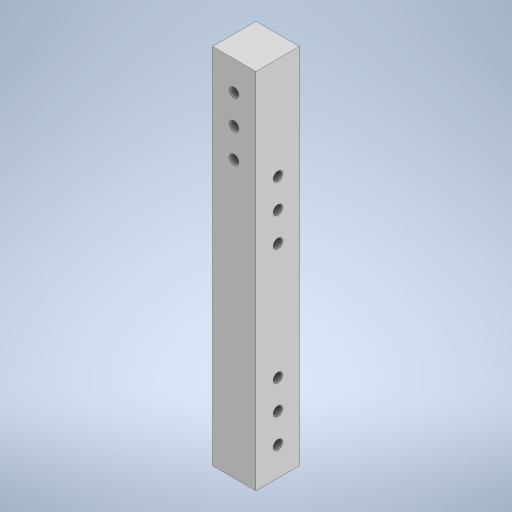
# Autodesk Inventor part: 射出_角柱11
Saved by Autodesk Inventor 2023 (Build 270158000, 158)
## iProperties
Created: 2022-04-20
Part Number: 射出_角柱11
Material: 一般
Document SubType Name: Modeling
Designer: yuta
Density: 1 g/cm^3
Appearance: 既定
Author: yuta
Autodesk Inventor part; units mm, degrees
ref_plane "YZ Plane" through (0, 0, 0) normal (1, 0, 0) x (0, 1, 0)
ref_plane "XZ Plane" through (0, 0, 0) normal (0, 1, 0) x (-1, 0, 0)
ref_plane "XY Plane" through (0, 0, 0) normal (0, 0, 1) x (1, 0, 0)
sketch "スケッチ1" plane through (0, 0, 0) normal (0, 1, 0) x (-1, 0, 0)
  line L0 (0, 0) -> (15, 0)
  line L1 (15, 0) -> (15, -15)
  line L2 (15, -15) -> (0, -15)
  line L3 (0, -15) -> (0, 0)
  dimension "d0" = 15
  dimension "d1" = 15
  constraints: 8 end point, 2 parallel, 1 horizontal, 1 perpendicular
  measures "d0" distance of L1.end L2.end
  measures "d1" distance of L0.end L1.end
extrude "押し出し1" add sketch "スケッチ1" along normal blind 125
sketch "スケッチ2" plane through (-15, 0, 0) normal (0, 0, 1) x (1, 0, 0)
  line L0 (0, 125) -> (15, 125) projected
  line L1 (0, 0) -> (0, 125) projected
  point P0 (15, 0)
  point P1 (7.5, 115)
  point P2 (7.5, 105)
  point P3 (7.5, 95)
  dimension "d4" = 10
  dimension "d5" = 7.5
  dimension "d6" = 7.5
  dimension "d7" = 7.5
  dimension "d8" = 10
  dimension "d9" = 10
  measures "d4" distance from line of L0 point (7.5, 115)
  measures "d5" distance from line of L1 point (7.5, 115)
  measures "d6" distance from line of L1 point (7.5, 105)
  measures "d7" distance from line of L1 point (7.5, 95)
  measures "d8" distance of point (7.5, 105) point (7.5, 115)
  measures "d9" distance of point (7.5, 95) point (7.5, 105)
hole "穴1" at (-7.5, 115, 0) at (-7.5, 105, 0) at (-7.5, 95, 0) direction (0, 0, -1) diameter 3.2 end through all
sketch "スケッチ3" plane through (0, 0, 0) normal (1, 0, 0) x (0, 0, -1)
  line L0 (0, 125) -> (15, 125) projected
  line L1 (15, 0) -> (15, 125) projected
  line L2 (0, 0) -> (15, 0) projected
  point P0 (7.5, 90)
  point P1 (7.5, 80)
  point P2 (7.5, 70)
  point P3 (7.5, 30)
  point P4 (7.5, 20)
  point P5 (7.5, 10)
  dimension "d17" = 35
  dimension "d18" = 7.5
  dimension "d19" = 10
  dimension "d20" = 10
  dimension "d21" = 30
  dimension "d22" = 7.5
  dimension "d23" = 7.5
  dimension "d24" = 7.5
  dimension "d25" = 10
  dimension "d26" = 10
  measures "d17" distance from line of L0 point (7.5, 90)
  measures "d18" distance from line of L1 point (7.5, 90)
  measures "d19" distance of point (7.5, 80) point (7.5, 90)
  measures "d20" distance of point (7.5, 70) point (7.5, 80)
  measures "d21" distance from line of L2 point (7.5, 30)
  measures "d22" distance from line of L1 point (7.5, 30)
  measures "d23" distance from line of L1 point (7.5, 20)
  measures "d24" distance from line of L1 point (7.5, 10)
  measures "d25" distance of point (7.5, 20) point (7.5, 30)
  measures "d26" distance of point (7.5, 10) point (7.5, 20)
hole "穴2" at (0, 90, -7.5) at (0, 80, -7.5) at (0, 70, -7.5) at (0, 30, -7.5) at (0, 20, -7.5) at (0, 10, -7.5) direction (-1, 0, 0) diameter 3.2 end through all
